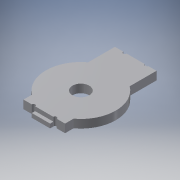
# Autodesk Inventor part: 付け根ロール_メインフレーム_1_1
Saved by Autodesk Inventor 2018 (Build 220112000, 112)
## iProperties
Created: 2016-05-01
Part Number: 付け根ロール_メインフレーム_1_1
Material: アルミニウム 2014-T4
Document SubType Name: Modeling
Designer: hiroaki
Density: 2.8 g/cm^3
Appearance: サテン
Mass: 15.1698 g
Surface Area: 53.0669 cm^2
Volume: 5.41778 cm^3
Author: hiroaki
Autodesk Inventor part; units mm, degrees
ref_plane "YZ Plane" through (0, 0, 0) normal (1, 0, 0) x (0, 1, 0)
ref_plane "XZ Plane" through (0, 0, 0) normal (0, 1, 0) x (-1, 0, 0)
ref_plane "XY Plane" through (0, 0, 0) normal (0, 0, 1) x (1, 0, 0)
derived "付け根ロール_基礎.ipt"
sketch "スケッチ1" plane through (0, 0, 0) normal (0, 0, 1) x (1, 0, 0)
  circle A0 centre (0, 0) radius 5.05 projected
  circle A1 centre (0, -8.5) radius 1.35 projected
  circle A2 centre (0, -8.5) radius 2.5 projected
  circle A3 centre (-5.6569, -5.6569) radius 1.55 projected
  line L0 (-5.6569, -5.6569) -> (0, 0) construction
  line L1 (0, 0) -> (0, -8.5) construction
  line L2 (-4.835, -8.7241) -> (-7.9022, -7.9022) construction
  line L3 (-7.9022, -7.9022) -> (-8.7241, -4.835) construction
  line L4 (-8.7241, -4.835) -> (-6.4787, -2.5896) construction
  line L5 (-6.4787, -2.5896) -> (-3.4115, -3.4115) construction
  line L6 (-3.4115, -3.4115) -> (-2.5896, -6.4787) construction
  line L7 (-2.5896, -6.4787) -> (-4.835, -8.7241) construction
  circle A4 centre (5.6569, -5.6569) radius 1.55 projected
  line L8 (8.7241, -4.835) -> (7.9022, -7.9022) construction
  line L9 (7.9022, -7.9022) -> (4.835, -8.7241) construction
  line L10 (4.835, -8.7241) -> (2.5896, -6.4787) construction
  line L11 (3.4115, -3.4115) -> (6.4787, -2.5896) construction
  line L12 (2.5896, -6.4787) -> (3.4115, -3.4115) construction
  line L13 (6.4787, -2.5896) -> (8.7241, -4.835) construction
  circle A5 centre (8.5, 0) radius 2.5 projected
  circle A6 centre (8.5, 0) radius 1.35 projected
  circle A7 centre (5.6569, 5.6569) radius 1.55 projected
  line L14 (4.835, 8.7241) -> (7.9022, 7.9022) construction
  line L15 (7.9022, 7.9022) -> (8.7241, 4.835) construction
  line L16 (8.7241, 4.835) -> (6.4787, 2.5896) construction
  line L17 (3.4115, 3.4115) -> (2.5896, 6.4787) construction
  line L18 (6.4787, 2.5896) -> (3.4115, 3.4115) construction
  line L19 (2.5896, 6.4787) -> (4.835, 8.7241) construction
  circle A8 centre (0, 8.5) radius 2.5 projected
  circle A9 centre (0, 8.5) radius 1.35 projected
  circle A10 centre (-5.6569, 5.6569) radius 1.55 projected
  line L20 (-8.7241, 4.835) -> (-7.9022, 7.9022) construction
  line L21 (-7.9022, 7.9022) -> (-4.835, 8.7241) construction
  line L22 (-4.835, 8.7241) -> (-2.5896, 6.4787) construction
  line L23 (-3.4115, 3.4115) -> (-6.4787, 2.5896) construction
  line L24 (-2.5896, 6.4787) -> (-3.4115, 3.4115) construction
  line L25 (-6.4787, 2.5896) -> (-8.7241, 4.835) construction
  circle A11 centre (-8.5, 0) radius 2.5 projected
  circle A12 centre (-8.5, 0) radius 1.35 projected
  circle A13 centre (0, 0) radius 12.45 construction
  circle A14 centre (0, 0) radius 21 construction
  line L26 (-12.5, 33) -> (-12.5, -22) construction
  line L27 (-12.5, -22) -> (-7.55, -22)
  line L28 (-12.5, 33) -> (-7.55, 33)
  line L29 (7.55, 33) -> (12.5, 33)
  line L30 (12.5, 33) -> (12.5, -22) construction
  line L31 (12.5, -22) -> (7.55, -22)
  line L32 (0, 0) -> (0, 8.5) construction
  line L33 (-5.5, 33.3202) -> (-5.5, 35)
  line L34 (-5.5, 35) -> (5.5, 35)
  line L35 (5.5, 35) -> (5.5, 33.3202)
  line L36 (-5.5, -22.3202) -> (-5.5, -24)
  line L37 (-5.5, -24) -> (5.5, -24)
  line L38 (5.5, -24) -> (5.5, -22.3202)
  arc A15 (-7.55, 33) -> (-5.5, 33.3202) centre (-6.5, 33) ccw
  line L39 (-7.55, 33) -> (-5.5, 33) construction
  line L40 (-5.5, 33.3202) -> (-5.5, 33.3202) construction
  arc A16 (5.5, 33.3202) -> (7.55, 33) centre (6.5, 33) ccw
  arc A17 (-5.5, -22.3202) -> (-7.55, -22) centre (-6.5, -22) ccw
  arc A18 (7.55, -22) -> (5.5, -22.3202) centre (6.5, -22) ccw
  line L41 (-11.05, 35) -> (-7.95, 35) construction
  line L42 (-7.95, 35) -> (-7.95, 31.6002) construction
  line L43 (-7.95, 31.6002) -> (-11.05, 31.6002) construction
  line L44 (-11.05, 31.6002) -> (-11.05, 35) construction
  line L45 (-9.5, 35) -> (-9.5, 31.6002) construction
  line L46 (12.5, 5.5) -> (-12.5, 5.5) construction
  line L47 (-12.5, -22) -> (-12.5, -16.8745)
  arc A19 (-12.5, 16.8745) -> (-12.5, -16.8745) centre (0, 0) ccw
  line L48 (-12.5, 16.8745) -> (-12.5, 33)
  line L49 (12.5, -22) -> (12.5, -16.8745)
  arc A20 (12.5, -16.8745) -> (12.5, 16.8745) centre (0, 0) ccw
  line L50 (12.5, 33) -> (12.5, 16.8745)
  circle A21 centre (0, 24.25) radius 3.25 construction
  circle A22 centre (0, 24.25) radius 1.05 projected
  circle A23 centre (-24.25, 0) radius 1.05 projected
  circle A24 centre (0, -24.25) radius 1.05 projected
  circle A25 centre (24.25, 0) radius 1.05 projected
  line L51 (2.75, 25.8377) -> (2.75, 22.6623) projected
  line L52 (2.75, 22.6623) -> (0, 21.0746) projected
  line L53 (0, 21.0746) -> (-2.75, 22.6623) projected
  line L54 (-2.75, 22.6623) -> (-2.75, 25.8377) projected
  line L55 (-2.75, 25.8377) -> (0, 27.4254) projected
  line L56 (0, 27.4254) -> (2.75, 25.8377) projected
  dimension "d22" = 1.05
  dimension "d23" = 25
  dimension "d24" = 55
  dimension "d25" = 2
  dimension "d26" = 2
  dimension "d27" = 22
  dimension "d28" = 7
  dimension "d29" = 3.1
  dimension "d30" = 3
  dimension "d49" = 3
  constraints: 50 end point, 15 point on circle, 9 perpendicular, 9 symmetric about line, 6 centre point, 5 collinear, 4 horizontal, 4 midpoint, 4 vertical, 3 parallel, 2 coincident, 1 equal radius, 1 point on line, 1 vertical alignment, 4 other
  measures "d22" radius of A15
  measures "d23" distance between parallel lines of L26 L30
  measures "d24" distance of L29.end L30.end
  measures "d25" distance between parallel lines of L29 L34
  measures "d26" distance between parallel lines of L37 L31
  measures "d27" distance from line of A14.centre L31
  measures "d28" distance between parallel lines of L33 L26
  measures "d29" distance of L41.start L41.end
  measures "d30" distance between parallel lines of L26 L45
  measures "d49" distance from line of L45 A15.centre
extrude "押し出し1" add sketch "スケッチ1" along normal blind 5 contours L47 A19 L48 L28 A15 L33 L34 L35 A16 L29 L50 A20 L49 L31 A18 L38 L37 A24 L36 A17 L27 | A24 L37 | A22 | L51 L52 L53 L54 L55 L56 picked at (0.0124, -23.6569)
sketch "スケッチ6" plane through (-5.5, -24, 5) normal (0, 0, 1) x (1, 0, 0)
  line L0 (-2.05, 57) -> (-7, 57) projected
  line L1 (-7, 2) -> (-2.05, 2) projected
  line L2 (-3.4142, -3.7238) -> (17.6304, -3.7238)
  line L3 (17.6304, -3.7238) -> (17.6304, 2)
  line L4 (17.6304, 2) -> (-3.4142, 2)
  line L5 (-3.4142, 2) -> (-3.4142, -3.7238)
  line L6 (-1.5604, 57) -> (14.161, 57)
  line L7 (14.161, 57) -> (14.161, 64.8853)
  line L8 (14.161, 64.8853) -> (-1.5604, 64.8853)
  line L9 (-1.5604, 64.8853) -> (-1.5604, 57)
  constraints: 16 end point, 4 parallel, 2 collinear, 2 horizontal, 2 perpendicular
extrude "押し出し3" cut sketch "スケッチ6" against normal blind 2.5
sketch "スケッチ11" plane through (7.55, -22, 5) normal (0, 0, 1) x (1, 0, 0)
  circle A0 centre (0.95, 22) radius 2.5 projected
  circle A1 centre (0.95, 22) radius 2.5
  circle A2 centre (-1.8931, 27.6569) radius 1.55 projected
  circle A3 centre (-1.8931, 27.6569) radius 1.55
  circle A4 centre (-7.55, 30.5) radius 2.5 projected
  circle A5 centre (-7.55, 30.5) radius 2.5
  circle A6 centre (-13.2069, 27.6569) radius 1.55 projected
  circle A7 centre (-13.2069, 27.6569) radius 1.55
  circle A8 centre (-16.05, 22) radius 2.5 projected
  circle A9 centre (-16.05, 22) radius 2.5
  circle A10 centre (-13.2069, 16.3431) radius 1.55 projected
  circle A11 centre (-13.2069, 16.3431) radius 1.55
  circle A12 centre (-7.55, 13.5) radius 2.5 projected
  circle A13 centre (-7.55, 13.5) radius 2.5
  circle A14 centre (-1.8931, 16.3431) radius 1.55 projected
  circle A15 centre (-1.8931, 16.3431) radius 1.55
  point P0 (-7.55, 22)
  constraints: 8 centre point, 8 coincident
extrude "押し出し8" add sketch "スケッチ11" against normal up to surface (5 mm away)
equation "\"d26\" = d25"
equation "\"d28\" = d17 + d18"
equation "\"d30\" = d17"
equation "\"d17\" = 3"
equation "\"d18\" = 4"
